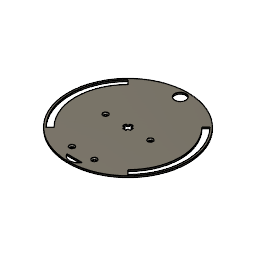
top2 (Autodesk Fusion 360 design; units mm, degrees)
Autodesk Fusion 360 part; units mm, degrees
sketch "Esboço1" plane through (0, 0, 0) normal (0, 1, 0) x (1, 0, 0)
  circle A0 centre (0, 0) radius 90
  dimension "d1" = 180
  constraint coincident A0.centre origin
  measures "d1" diameter of A0
sketch "Esboço2" plane through (0, 0, 0) normal (0, 1, 0) x (1, 0, 0)
  circle A0 centre (0, 0) radius 80
  line L0 (0, 0) -> (0, 80)
  line L1 (0, 0) -> (80, 0)
  line L2 (0, 0) -> (-80, 0)
  dimension "d2" = 160
  constraint coincident A0.centre L0.start
  constraint coincident A0 L0.end
  constraint vertical L0
  constraint coincident A0 L1.end
  constraint coincident A0 L2.end
  constraint perpendicular L0 L2
  measures "d2" diameter of A0
extrude "Extrusão1" add sketch "Esboço2" along normal blind 5
sketch "Esboço5" plane through (0, 10, 0) normal (0, 1, 0) x (-1, 0, 0)
  line L0 (-37.5, 82) -> (-37.5, 14.8926)
  line L1 (-37.5, 14.8926) -> (37.5, 14.8926)
  line L2 (37.5, 64.8926) -> (-37.5, 64.8926)
  line L3 (-37.5, 14.8926) -> (-37.5, 64.8926)
  line L4 (37.5, 64.8926) -> (37.5, 14.8926)
  line L5 (37.5, 14.8926) -> (-37.5, 14.8926)
  line L6 (37.5, 5.248) -> (37.5, 14.8926)
  line L7 (37.5, 5.248) -> (-37.6134, 5.248)
  line L8 (-37.6134, 5.248) -> (-37.5, 14.8926)
  line L9 (-37.5, 20.793) -> (37.5, 20.793)
  line L10 (37.5, 20.793) -> (37.5, 14.8926)
  dimension "d5" = 50
  constraint coincident L0 L2.end
  constraint perpendicular L0 L2
  constraint coincident L0.end L1.start
  constraint coincident L1.end L4.end
  constraint perpendicular L5 L6
  constraint perpendicular L6 L7
  constraint coincident L3 L9.start
  constraint coincident L4 L9.end
  constraint perpendicular L4 L9
  constraint perpendicular L5 L10
  measures "d5" distance of L2.start L1.end
extrude "Extrusão2" cut sketch "Esboço5" against normal blind 8 contours L0 L2 L3 L4 L9 | L0 L1 L3 L4 L5 L9 L10
sketch "Esboço8" plane through (0, 5, 0) normal (0, 1, 0) x (-1, 0, 0)
  line L0 (-37.5, 14.8926) -> (-37.5, 64.8926)
  line L1 (-37.5, 64.8926) -> (37.5, 64.8926)
  line L2 (37.5, 64.8926) -> (37.5, 14.8926)
  line L3 (37.5, 14.8926) -> (-37.5, 14.8926)
  circle A0 centre (0, 0) radius 80
  line L4 (1.0124, 14.8926) -> (1.0124, 14.6341)
  line L5 (-0.9835, 14.7615) -> (-0.9835, -53.7385)
  line L6 (-0.9835, -53.7385) -> (-55.4835, -53.7385)
  line L7 (-55.4835, -53.7385) -> (-55.4835, 14.7615)
  line L8 (-0.9835, 14.7615) -> (-55.4835, 14.7615)
  line L9 (0, 0) -> (0, 80)
  circle A1 centre (-52.2335, -50.4885) radius 1.5
  line L10 (-55.4835, 14.7615) -> (-55.4835, 11.5115)
  line L11 (-0.9835, -50.4885) -> (-0.9835, -53.7385)
  circle A2 centre (-4.2335, -50.4885) radius 1.5
  circle A3 centre (-4.2335, 11.5115) radius 1.5
  circle A4 centre (-52.2335, 11.5115) radius 1.5
  line L12 (55.4835, -53.7385) -> (55.4835, 14.7615)
  line L13 (0.9835, -53.7385) -> (55.4835, -53.7385)
  line L14 (0.9835, 14.7615) -> (0.9835, -53.7385)
  circle A5 centre (4.2335, 11.5115) radius 1.5
  line L15 (0.9835, 14.7615) -> (55.4835, 14.7615)
  circle A6 centre (52.2335, 11.5115) radius 1.5
  circle A7 centre (52.2335, -50.4885) radius 1.5
  circle A8 centre (4.2335, -50.4885) radius 1.5
  point P0 (-28.2335, -19.4885)
  dimension "d12" = 68.5
  dimension "d13" = 54.5
  dimension "d17" = 3
  dimension "d18" = 3.25
  dimension "d20" = 3
  dimension "d21" = 3
  dimension "d22" = 3
  constraint vertical L4
  constraint perpendicular L5 L6
  constraint perpendicular L6 L7
  constraint perpendicular L7 L8
  constraint coincident L3 L4.start
  constraint perpendicular L8 L10
  constraint coincident L5 L11.start
  constraint symmetric L5.start L9 L14.start
  constraint symmetric L5.end L9 L13.start
  constraint symmetric L6.end L9 L12.start
  constraint symmetric L7.end L9 L12.end
  constraint symmetric L9 A1 A7
  constraint symmetric L9 A2 A8
  constraint symmetric L9 A3 A5
  constraint symmetric L9 A4 A6
  measures "d12" distance of L5.start L5.end
  measures "d13" distance of L5.end L6.end
  measures "d17" diameter of A1
  measures "d18" distance of L7.end L10.end
  measures "d20" diameter of A2
  measures "d21" diameter of A3
  measures "d22" diameter of A4
extrude "Extrusão3" cut sketch "Esboço8" against normal blind 3 contours L5 L6 L7 L8 L10 L11 | A1 | A2 | A3 | A4 | L12 L13 L14 L15 | A5 | A6 | A7 | A8
extrude "Extrusão4" cut sketch "Esboço5" against normal blind 8 contours L0 L1 L3 L4 L5 L9 L10 | L1 L5 L6 L7 L8
sketch "Esboço9" plane through (0, 5, 0) normal (0, 1, 0) x (-1, 0, 0)
  line L0 (0.9835, 5.248) -> (-0.9835, 5.248)
  line L1 (-0.9835, 5.248) -> (-0.9835, -53.7385)
  line L2 (-0.9835, -53.7385) -> (-55.4835, -53.7385)
  line L3 (-55.4835, -53.7385) -> (-55.4835, 14.7615)
  line L4 (-55.4835, 14.7615) -> (-37.5015, 14.7615)
  line L5 (-37.5015, 14.7615) -> (-37.5, 14.8926)
  line L6 (-37.5, 14.8926) -> (-37.5, 64.8926)
  line L7 (-37.5, 64.8926) -> (37.5, 64.8926)
  line L8 (37.5, 64.8926) -> (37.5, 14.7615)
  line L9 (37.5, 14.7615) -> (55.4835, 14.7615)
  line L10 (55.4835, 14.7615) -> (55.4835, -53.7385)
  line L11 (55.4835, -53.7385) -> (0.9835, -53.7385)
  line L12 (0.9835, -53.7385) -> (0.9835, 5.248)
  circle A0 centre (0, 0) radius 80
  line L13 (60, -25) -> (60, 10)
  line L14 (70, 10) -> (60, 10)
  line L15 (70, 10) -> (70, -25)
  line L16 (60, -25) -> (70, -25)
  circle A1 centre (0, 71.8926) radius 5
  line L17 (0, 0) -> (0, -80)
  line L18 (-60, -25) -> (-70, -25)
  line L19 (-70, 10) -> (-70, -25)
  line L20 (-60, -25) -> (-60, 10)
  line L21 (-70, 10) -> (-60, 10)
  line L22 (41, 24.7536) -> (41, 58.1605)
  line L23 (41, 58.1605) -> (46, 58.1605)
  line L24 (46, 58.1605) -> (46, 48.1605)
  line L25 (41, 24.7536) -> (46, 24.7536)
  line L26 (-41, 24.7536) -> (-45.5, 24.7536)
  line L27 (-41, 24.7536) -> (-41, 58.1605)
  line L28 (-41, 58.1605) -> (-45.5, 58.1605)
  line L29 (46, 58.1605) -> (46, 48.1605)
  line L30 (46, 48.1605) -> (53, 48.1605)
  line L31 (53, 48.1605) -> (53, 24.7536)
  line L32 (46, 24.7536) -> (53, 24.7536)
  line L33 (-46, 48.1605) -> (-53, 48.1605)
  line L34 (-46, 58.1605) -> (-46, 48.1605)
  line L35 (-53, 48.1605) -> (-53, 24.7536)
  line L36 (-41, 58.1605) -> (-46, 58.1605)
  line L37 (-53, 24.7536) -> (-41, 24.7536)
  dimension "d31" = 10
  dimension "d35" = 5
  dimension "d46" = 10
  dimension "d47" = 7
  constraint perpendicular L13 L14
  constraint perpendicular L14 L15
  constraint perpendicular L13 L16
  constraint symmetric L13.end L17 L20.end
  constraint symmetric L14.start L17 L19.start
  constraint symmetric L15.end L17 L18.end
  constraint symmetric L13.start L17 L18.start
  constraint perpendicular L22 L23
  constraint perpendicular L23 L24
  constraint perpendicular L24 L25
  constraint perpendicular L23 L29
  constraint perpendicular L24 L30
  constraint perpendicular L30 L31
  constraint perpendicular L31 L32
  constraint symmetric L17 L22.end L27.end
  constraint symmetric L17 L23.end L34.start
  constraint symmetric L17 L24.end L33.start
  constraint symmetric L17 L30.end L33.end
  constraint symmetric L17 L31.end L35.end
  constraint perpendicular L27 L37
  measures "d31" diameter of A1
  measures "d35" distance of L22.end L23.end
  measures "d46" distance of L23.end L24.end
  measures "d47" distance of L24.end L30.end
extrude "Extrusão5" cut sketch "Esboço9" against normal blind 45 contours L13 L14 L15 L16 | A1 | L18 L19 L20 L21 | L22 L23 L24 L25 L29 L30 L31 L32
sketch "Esboço10" plane through (0, 0, 0) normal (0, -1, 0) x (1, 0, 0)
  circle A0 centre (0, 71.8926) radius 5
  line L0 (-41, 24.7536) -> (-53, 24.7536)
  line L1 (-46, 48.1605) -> (-46, 58.1605)
  line L2 (-46, 58.1605) -> (-41, 58.1605)
  line L3 (-41, 58.1605) -> (-41, 24.7536)
  line L4 (-60, 10) -> (-60, -25)
  line L5 (-60, -25) -> (-70, -25)
  line L6 (-70, -25) -> (-70, 10)
  line L7 (-70, 10) -> (-60, 10)
  line L8 (60, 10) -> (70, 10)
  line L9 (70, 10) -> (70, -25)
  line L10 (70, -25) -> (60, -25)
  line L11 (60, -25) -> (60, 10)
  circle A1 centre (0, 0) radius 80
  circle A2 centre (0, 0) radius 67.5 construction
  line L12 (0, 0) -> (0, 67.5) construction
  line L13 (0, 67.5) -> (0, 60)
  line L14 (0, 60) -> (-15, 60) construction
  circle A3 centre (-15, 60) radius 1.4
  circle A4 centre (15, 60) radius 1.4
  line L15 (0, 0) -> (-30, 0) construction
  circle A5 centre (-30, 0) radius 1.4
  circle A6 centre (30, 0) radius 1.4
  line L16 (-53, 24.7536) -> (-53, 48.1605)
  line L17 (-53, 48.1605) -> (-46, 48.1605)
  dimension "d38" = 135
  dimension "d39" = 7.5
  dimension "d40" = 15
  dimension "d41" = 2.8
  dimension "d42" = 30
  dimension "d43" = 2.8
  constraint coincident A1.centre A2.centre
  constraint coincident A2 L12.end
  constraint vertical L12
  constraint parallel L12 L13
  constraint perpendicular L13 L14
  constraint coincident L14.end A3.centre
  constraint symmetric L12 A3 A4
  constraint perpendicular L12 L15
  constraint coincident L15.end A5.centre
  constraint symmetric L12 A5 A6
  measures "d38" diameter of A2
  measures "d39" distance of L12.end L13.end
  measures "d40" distance of L13.end L14.end
  measures "d41" diameter of A3
  measures "d42" distance of A1.centre L15.end
  measures "d43" diameter of A5
extrude "Extrusão6" cut sketch "Esboço10" against normal blind 15 contours A3 | A4 | A5 | A6
extrude "Extrusão7" cut sketch "Esboço9" against normal blind 15 contours L26 L27 L28 L33 L34 L35 L36 L37
extrude "Extrusão8" cut 1 faces at (-32.1557, 5, -58.9197) along direction (0, -1, 0) blind 2.5
extrude "Extrusão9" cut 1 faces at (-32.1557, 2.5, -58.9197) along direction (0, -1, 0) blind 0.5
sketch "Esboço11" plane through (0, 2, 0) normal (0, 1, 0) x (-1, 0, 0)
  circle A0 centre (0, 0) radius 80
  line L0 (-70, 10) -> (-60, 10)
  line L1 (-60, 10) -> (-60, -25)
  line L2 (-60, -25) -> (-70, -25)
  line L3 (-70, -25) -> (-70, 10)
  line L4 (60, -25) -> (60, 10)
  line L5 (60, 10) -> (70, 10)
  line L6 (70, 10) -> (70, -25)
  line L7 (70, -25) -> (60, -25)
  circle A1 centre (0, 71.8926) radius 5
  line L8 (53, 48.1605) -> (53, 24.7536)
  line L9 (53, 24.7536) -> (41, 24.7536)
  line L10 (41, 24.7536) -> (41, 58.1605)
  line L11 (41, 58.1605) -> (46, 58.1605)
  line L12 (46, 58.1605) -> (46, 48.1605)
  line L13 (46, 48.1605) -> (53, 48.1605)
  line L14 (-41, 58.1605) -> (-41, 24.7536)
  line L15 (-41, 24.7536) -> (-53, 24.7536)
  line L16 (-53, 24.7536) -> (-53, 48.1605)
  line L17 (-53, 48.1605) -> (-46, 48.1605)
  line L18 (-46, 48.1605) -> (-46, 58.1605)
  line L19 (-46, 58.1605) -> (-41, 58.1605)
  circle A2 centre (-15, 60) radius 1.4
  circle A3 centre (30, 0) radius 1.4
  circle A4 centre (15, 60) radius 1.4
  circle A5 centre (-30, 0) radius 1.4
  line L20 (-60, -25) -> (-60, -35)
  line L21 (-70, -25) -> (-70, -30)
  line L22 (-70, -30) -> (-65, -35)
  line L23 (-65, -35) -> (-60, -35)
  line L24 (-46, 24.7536) -> (-41, 24.7536)
  line L25 (-41, 24.7536) -> (-41, 58.1605)
  line L26 (-46, 58.1605) -> (-41, 58.1605)
  line L27 (-46, 58.1605) -> (-46, 48.1605)
  line L28 (-53, 48.1605) -> (-46, 48.1605)
  line L29 (-53, 48.1605) -> (-53, 24.7536)
  line L30 (-46, 24.7536) -> (-53, 24.7536)
  line L31 (0, 0) -> (0, 16.0765) construction
  line L32 (46, 58.1605) -> (46, 48.1605)
  line L33 (46, 58.1605) -> (41, 58.1605)
  line L34 (41, 24.7536) -> (41, 58.1605)
  line L35 (46, 24.7536) -> (41, 24.7536)
  line L36 (46, 24.7536) -> (53, 24.7536)
  line L37 (53, 48.1605) -> (53, 24.7536)
  line L38 (53, 48.1605) -> (46, 48.1605)
  line L39 (60, -25) -> (60, -35)
  line L40 (65, -35) -> (60, -35)
  line L41 (70, -30) -> (65, -35)
  line L42 (70, -25) -> (70, -30)
  line L43 (60, -25) -> (70, -25)
  dimension "d54" = 10
  constraint coincident L1.end L2.start
  constraint perpendicular L2 L20
  constraint coincident L2.end L3.start
  constraint perpendicular L2 L21
  constraint perpendicular L20 L23
  constraint coincident L17.end L18.start
  constraint coincident L15 L24.start
  constraint coincident L14.end L15.start
  constraint coincident L14.start L19.end
  constraint coincident L18.end L19.start
  constraint coincident L16.end L17.start
  constraint coincident L15.end L16.start
  constraint coincident A0.centre L31.start
  constraint vertical L31
  constraint symmetric L1.end L31 L4.start
  constraint symmetric L2.end L31 L6.end
  constraint symmetric L20.end L31 L39.end
  constraint symmetric L21.end L31 L41.start
  constraint symmetric L22.end L31 L40.start
  constraint symmetric L17.end L31 L12.end
  constraint symmetric L24.start L31 L35.start
  constraint symmetric L14.end L31 L9.end
  constraint symmetric L14.start L31 L10.end
  constraint symmetric L18.end L31 L11.end
  constraint symmetric L16.end L31 L8.start
  constraint symmetric L15.end L31 L8.end
  measures "d54" distance of L1.end L20.end
extrude "Extrusão10" add sketch "Esboço11" against normal blind 2 contours L8 L9 L10 L11 L12 L13 L32 L33 L34 L35 L36 L37 L38 | L14 L15 L16 L17 L18 L19 L24 L25 L26 L27 L28 L29 L30
extrude "Extrusão11" cut sketch "Esboço11" against normal blind 10 contours L2 L20 L21 L22 L23 | L7 L39 L40 L41 L42 L43
sketch "Esboço12" plane through (0, 2, 0) normal (0, 1, 0) x (-1, 0, 0)
  circle A0 centre (-30, 0) radius 1.4
  circle A1 centre (15, 60) radius 1.4
  circle A2 centre (30, 0) radius 1.4
  circle A3 centre (-15, 60) radius 1.4
  circle A4 centre (0, 71.8926) radius 5
  line L0 (70, 10) -> (70, -30)
  line L1 (70, -30) -> (65, -35)
  line L2 (65, -35) -> (60, -35)
  line L3 (60, -35) -> (60, 10)
  line L4 (60, 10) -> (70, 10)
  circle A5 centre (0, 0) radius 80
  line L5 (-70, -30) -> (-70, 10)
  line L6 (-70, 10) -> (-60, 10)
  line L7 (-60, 10) -> (-60, -35)
  line L8 (-60, -35) -> (-65, -35)
  line L9 (-65, -35) -> (-70, -30)
  line L10 (0, 0) -> (0, 80) construction
  line L11 (65, -35) -> (70, -30)
  line L12 (0, 0) -> (0, -80) construction
  line L13 (0, -80) -> (0, -70) construction
  circle A6 centre (0, -70) radius 7.5
  circle A7 centre (0, 0) radius 77.5
  line L14 (0, 0) -> (-70, 33.2603)
  line L15 (-70, 33.2603) -> (-60.9677, 28.9687)
  circle A8 centre (0, 0) radius 67.5
  line L16 (0, 0) -> (-16.8189, 0) construction
  line L17 (0, 0) -> (-70, -33.2603)
  dimension "d66" = 10
  dimension "d67" = 15
  dimension "d73" = 155
  dimension "d74" = 10
  constraint coincident A5.centre L10.start
  constraint coincident A5 L10.end
  constraint vertical L10
  constraint symmetric L5.start L10 L0.end
  constraint symmetric L8.end L10 L1.end
  constraint coincident A5 L12.end
  constraint parallel L10 L12
  constraint parallel L12 L13
  constraint coincident L13.end A6.centre
  constraint coincident A7 L14.end
  constraint parallel L14 L15
  constraint coincident L15.end A8
  constraint perpendicular L10 L16
  constraint symmetric A5.centre L16 L10.start
  constraint symmetric L14.end L16 L17.end
  measures "d66" distance of L12.end L13.end
  measures "d67" diameter of A6
  measures "d73" diameter of A7
  measures "d74" distance of L14.end L15.end
extrude "Extrusão12" add sketch "Esboço12" against normal blind 2 contours L3 L4 A8 | L0 L1 L2 L3 L4 L11 A8 | L5 L6 L9 A8 L17 | L6 L7 A8 L17 | L7 A8 L17 | L7 L8 L9 A8 L17
extrude "Extrusão13" cut sketch "Esboço12" against normal blind 20 contours A4 L0 L1 L2 L3 L4 L11 A6 A7 L14 L15 A8 | L5 L6 L9 A7 L14 L15 A8 L17 | L0 L1 L2 L3 L4 L11 A8 | L5 L6 L9 A8 L17 | A6 A8 | A6 A8
extrude "Extrusão14" add sketch "Esboço12" against normal blind 2 contours A0 | A1 | A2 | A3 | A4 L0 L1 L2 L3 L4 L11 A6 A7 L14 L15 A8 | A4 A8 | A4 L3 L4 L7 A6 L14 A8 L17 | L6 L7 L14 A8 L17 | L3 L4 A8 | L0 L1 L2 L3 L4 L11 A8 | L5 L6 L9 A8 L17 | L6 L7 A8 L17 | L7 A8 L17 | L7 L8 L9 A8 L17 | A6 A8 picked at (-0.1145, 67.2985) picked at (0, -65.8069)
extrude "Extrusão15" add sketch "Esboço12" against normal blind 2 contours L5 L6 L9 A7 L14 L15 A8 L17
extrude "Extrusão16" cut sketch "Esboço12" against normal blind 2 contours A6 A8 picked at (0, -65.8069)
extrude "Extrusão17" cut sketch "Esboço12" against normal blind 4 contours A4 A8 picked at (-0.1145, 67.2985)
sketch "Esboço13" plane through (0, 2, 0) normal (0, 1, 0) x (-1, 0, 0)
  circle A0 centre (0, 71.8926) radius 5
  circle A1 centre (0, -70) radius 7.5
  circle A2 centre (0, 0) radius 80
  circle A3 centre (0, 0) radius 77.5
  line L0 (0, 0) -> (54.8008, -54.8008)
  line L1 (0, 0) -> (77.5, 0) construction
  line L2 (0, 0) -> (54.8008, 54.8008)
  circle A4 centre (0, 0) radius 70
  line L3 (0, 0) -> (0, -19.0761) construction
  line L4 (0, 0) -> (-54.8008, -54.8008)
  line L5 (0, 0) -> (-54.8008, 54.8008)
  dimension "d83" = 155
  dimension "d84" = 45
  dimension "d86" = 140
  constraint coincident A2.centre A3.centre
  constraint horizontal L1
  constraint symmetric A2.centre L1 A3.centre
  constraint symmetric L0.end L1 L2.end
  constraint concentric A3 A4
  constraint perpendicular L1 L3
  constraint symmetric A2.centre L3 A3.centre
  constraint symmetric L0.end L3 L4.end
  constraint symmetric L2.end L3 L5.end
  measures "d83" diameter of A3
  measures "d84" angle of L0 L1
  measures "d86" diameter of A4
extrude "Extrusão18" cut sketch "Esboço13" against normal blind 35 contours A3 A4 L4 L5 | A3 L0 L2 A4
extrude "Extrusão19" cut sketch "Esboço10" against normal blind 15 contours A3 | A4 | A5 | A6
chamfer "Chanfro1" distance 2 angle 45 4 edges at (-31.3053, 2, -0.5063) (28.6947, 2, -0.5063) (-16.3053, 2, 59.4937) (13.6947, 2, 59.4937)
sketch "Esboço14" plane through (0, 2, 0) normal (0, 1, 0) x (-1, 0, 0)
  circle A0 centre (15, 60) radius 3.4
  circle A1 centre (30, 0) radius 3.4
  line L0 (49.4975, 49.4975) -> (54.8008, 54.8008)
  arc A2 (54.8008, -54.8008) -> (54.8008, 54.8008) centre (0, 0) ccw
  line L1 (54.8008, -54.8008) -> (49.4975, -49.4975)
  arc A3 (49.4975, -49.4975) -> (49.4975, 49.4975) centre (0, 0) ccw
  arc A4 (-54.8008, 54.8008) -> (-54.8008, -54.8008) centre (0, 0) ccw
  line L2 (-54.8008, 54.8008) -> (-49.4975, 49.4975)
  arc A5 (-49.4975, 49.4975) -> (-49.4975, -49.4975) centre (0, 0) ccw
  line L3 (-49.4975, -49.4975) -> (-54.8008, -54.8008)
  circle A6 centre (0, 71.8926) radius 5
  circle A7 centre (0, -70) radius 7.5
  circle A8 centre (0, 0) radius 80
  circle A9 centre (-30, 0) radius 3.4
  circle A10 centre (-15, 60) radius 3.4
  line L4 (0, -5) -> (0, -80) construction
  line L5 (0, -5) -> (2, -5)
  line L6 (2, 5) -> (0, 5)
  line L7 (0, 5) -> (-2, 5)
  line L8 (0, -5) -> (-2, -5)
  line L9 (5, 0) -> (5, -2)
  line L10 (5, 0) -> (5, 2)
  line L11 (-5, 2) -> (-5, -2)
  line L12 (2, -5) -> (2, -2)
  line L13 (2, 2) -> (2, 5)
  line L14 (-5, -2) -> (-2, -2)
  line L15 (2, -2) -> (5, -2)
  line L16 (-2, 5) -> (-2, 2)
  line L17 (-2, -2) -> (-2, -5)
  line L18 (0, 0) -> (0, 2) construction
  line L19 (0, 5) -> (0, 80) construction
  line L20 (5, 2) -> (2, 2)
  line L21 (-2, 2) -> (-5, 2)
  line L22 (0, 71.8926) -> (-10, 71.8926)
  line L23 (0, 71.8926) -> (10, 71.8926)
  line L24 (0, 80) -> (0, 78)
  arc A11 (10, 71.8926) -> (-10, 71.8926) centre (0, 66.7595) ccw
  dimension "d92" = 5
  dimension "d93" = 5
  dimension "d96" = 2
  dimension "d97" = 10
  dimension "d98" = 2
  dimension "d100" = 10
  dimension "d101" = 2
  dimension "d102" = 2
  dimension "d103" = 10
  dimension "d104" = 4
  dimension "d105" = 10
  dimension "d106" = 10
  dimension "d107" = 2
  constraint coincident A8 L4.end
  constraint vertical L4
  constraint coincident A2.centre A3.centre
  constraint coincident A8 L19.end
  constraint parallel L4 L18
  constraint perpendicular L4 L5
  constraint perpendicular L5 L12
  constraint perpendicular L6 L18
  constraint perpendicular L16 L20
  constraint coincident L12.end L14
  constraint collinear L12 L13
  constraint collinear L14 L15
  constraint coincident L14.end L16
  constraint coincident L16.end L20
  constraint collinear L16 L17
  constraint collinear L18 L19
  constraint collinear L20 L21
  constraint coincident A6.centre L22.start
  constraint perpendicular L19 L22
  constraint perpendicular L19 L23
  constraint parallel L19 L24
  constraint coincident L24.end A11
  measures "d92" distance of A2.centre L4.start
  measures "d93" distance of A2.centre L6.end
  measures "d96" distance of L4.start L5.end
  measures "d97" distance of L5.end L6.start
  measures "d98" distance of L6.start L6.end
  measures "d100" distance of L7.end L8.end
  measures "d101" distance of L9.start L9.end
  measures "d102" distance of L9.start L10.end
  measures "d103" distance of L10.end L11.start
  measures "d104" distance of L11.start L11.end
  measures "d105" distance of A6.centre L22.end
  measures "d106" distance of A6.centre L23.end
  measures "d107" distance of L19.end L24.end
extrude "Extrusão20" add sketch "Esboço14" against normal blind 2 contours A6 L22 L23 picked at (3.3147, 71.6442)
extrude "Extrusão21" cut sketch "Esboço14" against normal blind 13 contours A6 L22 L23 A11
extrude "Extrusão22" cut sketch "Esboço14" against normal blind 28 contours L5 L6 L7 L8 L9 L10 L11 L12 L13 L14 L15 L16 L17 L20 L21
extrude "Extrusão23" cut 5 faces at (-18.2125, 0, -39.2288) (31.3567, 0.0003, 0.3455) (-28.6433, 0.0003, 0.3455) (16.3983, 0.0001, 60.0698) (-13.6017, 0.0001, 60.0698) along direction (0, 1, 0) blind 0.5
extrude "Extrusão24" add 1 faces at (-27.295, 0.5, -38.1436) along direction (0, -1, 0) blind 0.5
